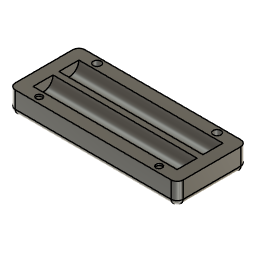
Cigar Box v1 (Autodesk Fusion 360 design; units mm, degrees)
Autodesk Fusion 360 part; units mm, degrees
sketch "Cigar Box" plane through (0, 0, 0) normal (0, 0, 1) x (1, 0, 0)
  line L0 (88.9, 36.875) -> (-88.9, 36.875)
  line L1 (-88.9, 36.875) -> (-88.9, -36.875)
  line L2 (-88.9, -36.875) -> (88.9, -36.875)
  line L3 (88.9, -36.875) -> (88.9, 36.875)
  line L4 (88.9, 36.875) -> (-88.9, -36.875) construction
  line L5 (-88.9, 36.875) -> (88.9, -36.875) construction
  line L6 (76.2, 24.175) -> (-76.2, 24.175)
  line L7 (-76.2, 24.175) -> (-76.2, 3.175)
  line L8 (-76.2, 3.175) -> (76.2, 3.175)
  line L9 (76.2, 3.175) -> (76.2, 24.175)
  line L10 (76.2, 24.175) -> (-76.2, 3.175) construction
  line L11 (-76.2, 24.175) -> (76.2, 3.175) construction
  line L12 (-76.2, 13.675) -> (76.2, 13.675)
  circle A0 centre (-63.5, 30.8) radius 4.075
  line L13 (-63.5, 30.8) -> (-63.5, 34.875) construction
  line L14 (-63.5, 34.875) -> (-63.5, 36.875) construction
  circle A1 centre (-63.5, -30.525) radius 3.375
  point P0 (0, 13.675)
  dimension "d1" = 177.8
  dimension "d3" = 152.4
  dimension "d4" = 21
  dimension "d5" = 3.175
  dimension "d6" = 8.15
  dimension "d7" = 2
  dimension "d8" = 25.4
  dimension "d9" = 12.7
  dimension "d10" = 6.75
  dimension "d11" = 6.35
  dimension "d12" = 25.4
  constraint horizontal L0
  constraint perpendicular L0 L1
  constraint parallel L0 L2
  constraint parallel L1 L3
  constraint coincident L4 origin
  constraint coincident L5 origin
  constraint horizontal L6
  constraint perpendicular L6 L7
  constraint parallel L6 L8
  constraint parallel L7 L9
  constraint coincident L10 P0
  constraint coincident L11 P0
  constraint vertical origin P0
  constraint midpoint L7 L12.start
  constraint midpoint L9 L12.end
  constraint coincident A0.centre L13.start
  constraint coincident A0 L13.end
  constraint vertical L13
  constraint coincident L0 L14.end
  constraint perpendicular L0 L14
  measures "d1" distance of L1.end L2.end
  measures "d3" distance of L7.end L8.end
  measures "d4" distance of L6.end L7.end
  measures "d5" distance of origin L8
  measures "d6" diameter of A0
  measures "d7" distance of L13.end L14.end
  measures "d8" distance of L1 A0.centre
  measures "d9" distance of L0 L6
  measures "d10" diameter of A1
  measures "d11" distance of L2 A1.centre
  measures "d12" distance of L1 A1.centre
extrude "Extrude1" add sketch "Cigar Box" against normal blind 24.13 contours L0 L1 L2 L3 | L6 L7 L9 L12 | L7 L8 L9 L12 | A0 | A1
extrude "Extrude2" cut sketch "Cigar Box" against normal blind 9 contours A0
extrude "Extrude3" cut sketch "Cigar Box" against normal blind 1.8 contours A1
mirror "Mirror1" about plane through (0, 0, 0) normal (1, 0, 0) of "Extrude2", "Extrude3"
revolve "Revolve1" cut sketch "Cigar Box" angle 360 about axis through (-76.2, 13.675, 0) along (1, 0, 0) contours L6 L7 L9 L12
mirror "Mirror2" about plane through (0, 0, 0) normal (0, 1, 0) of "Revolve1"
fillet "Fillet1" radius 6.35 4 edges at (88.9, -36.875, -12.065) (88.9, 36.875, -12.065) (-88.9, 36.875, -12.065) (-88.9, -36.875, -12.065)
fillet "Fillet1" radius 6.35 1 faces at (29.6333, -12.2917, -24.13)
named bodies: "Cigar Box"
